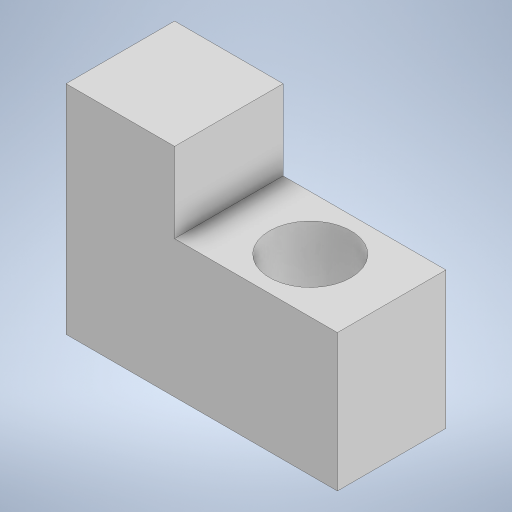
# Autodesk Inventor part: Cylinder Block
Saved by Autodesk Inventor 2023 (Build 270158000, 158)
## iProperties
Created: 2023-03-09
Part Number: Cylinder Block
Material: Generic
Document SubType Name: Modeling
Designer: tommy
Density: 1 g/cm^3
Appearance: Default
Author: tommy
Autodesk Inventor part; units mm, degrees
ref_plane "YZ Plane" through (0, 0, 0) normal (1, 0, 0) x (0, 1, 0)
ref_plane "XZ Plane" through (0, 0, 0) normal (0, 1, 0) x (-1, 0, 0)
ref_plane "XY Plane" through (0, 0, 0) normal (0, 0, 1) x (1, 0, 0)
sketch "Sketch1" plane through (0, 0, 0) normal (0, 1, 0) x (-1, 0, 0)
  line L0 (0, 0) -> (-76.2, 0)
  line L1 (-76.2, 0) -> (-76.2, 50.8)
  line L2 (-76.2, 50.8) -> (0, 50.8)
  line L3 (0, 50.8) -> (0, 0)
  line L4 (0, 50.8) -> (50.8, 50.8)
  line L5 (50.8, 50.8) -> (50.8, 0)
  line L6 (50.8, 0) -> (0, 0)
  line L7 (0, 0) -> (0, 50.8)
  circle A0 centre (-38.1, 25.4) radius 19.05
  circle A1 centre (25.4, 37.0829) radius 6.964
  line L8 (50.8, 25.4) -> (-76.2, 25.4)
  point P0 (-57.15, 25.4)
  point P1 (-19.05, 25.4)
  point P2 (0, 25.4)
  dimension "d0" = 76.2
  dimension "d1" = 50.8
  dimension "d2" = 50.8
  dimension "d3" = 38.1
  constraints: 18 end point, 4 parallel, 2 centre point, 2 horizontal, 2 midpoint, 2 perpendicular, 1 point on line
  measures "d0" distance of L1.end L2.end
  measures "d1" distance of L0.end L1.end
  measures "d2" distance of L5.end L6.end
  measures "d3" diameter of A0
extrude "Extrusion3" add sketch "Sketch1" along normal blind 64.2112 contours L8 A0 L1 L2 L3
extrude "Extrusion4" add sketch "Sketch1" along normal blind 101.6 contours L3 L4 L5 L8 | A1
mirror "Mirror1" about plane through (76.2, 0, 25.4) normal (0, 0, -1)
body "Solid1"
